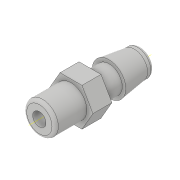
# Autodesk Inventor part: Suction_electrode_cap_side_dk
Saved by Autodesk Inventor 2020 (Build 240168000, 168)
## iProperties
Created: 2020-05-16
Part Number: Suction_electrode_cap_side_dk
Material: Generic
Document SubType Name: Modeling
Designer: Huai-Ti Lin
Density: 1 g/cm^3
Appearance: Default
Author: Huai-Ti Lin
Autodesk Inventor part; units mm, degrees
ref_plane "YZ Plane" through (0, 0, 0) normal (1, 0, 0) x (0, 1, 0)
ref_plane "XZ Plane" through (0, 0, 0) normal (0, 1, 0) x (-1, 0, 0)
ref_plane "XY Plane" through (0, 0, 0) normal (0, 0, 1) x (1, 0, 0)
sketch "Sketch1" plane through (0, 0, 0) normal (0, 1, 0) x (-1, 0, 0)
  line L0 (-1.05, 0) -> (-2.5, 0)
  line L1 (-2.5, 0) -> (-2.5, -5)
  line L2 (-2.5, -5) -> (-2.1, -5)
  line L3 (-2.1, -5) -> (-2.1, -16)
  line L4 (-2.1, -16) -> (-1.05, -16)
  line L5 (0, -19.2) -> (0, 3.2) projected
  line L6 (-1.05, 0) -> (-1.05, -16)
  line L7 (-2.1, -11) -> (-2.65, -11)
  line L8 (-2.65, -11) -> (-2.1, -15)
  point P0 (0, 0)
  dimension "d0" = 11
  dimension "d1" = 5
  dimension "d3" = 1.05
  dimension "d4" = 2.5
  dimension "d14" = 2.1
  dimension "d15" = 2.65
  dimension "d19" = 1
  dimension "d20" = 4
  constraints: 17 end point, 5 perpendicular, 2 point on line, 1 horizontal, 1 horizontal alignment
  measures "d0" distance of L2.end L3.end
  measures "d1" distance between parallel lines of L2 L0
  measures "d3" distance between parallel lines of L5 L6
  measures "d4" distance between parallel lines of L5 L1
  measures "d14" distance between parallel lines of L5 L3
  measures "d15" distance from line of L5 L7.end
  measures "d19" distance from line of L4 L8.end
  measures "d20" distance from line of L8.end L7
revolve "Revolution1" add sketch "Sketch1" angle 360 about axis through (0, 0, -10) along (0, 0, 1)
fillet "Fillet2" radius 0.5 2 edges at (-2.5, 0, 0) (-2.1, 0, -16)
sketch "Sketch3" plane through (0, 0, -5) normal (0, 0, -1) x (-1, 0, 0)
  line L0 (3.4641, 0) -> (1.7321, -3)
  line L1 (1.7321, -3) -> (-1.7321, -3)
  line L2 (-1.7321, -3) -> (-3.4641, 0)
  line L3 (-3.4641, 0) -> (-1.7321, 3)
  line L4 (-1.7321, 3) -> (1.7321, 3)
  line L5 (1.7321, 3) -> (3.4641, 0)
  circle A0 centre (0, 0) radius 1.05
  dimension "d21" = 6
  constraints: 12 end point, 2 coincident, 1 centre point, 13 other
  measures "d21" distance between parallel lines of L1 L4
extrude "Extrusion2" add sketch "Sketch3" along normal blind 3
body "Solid1"
